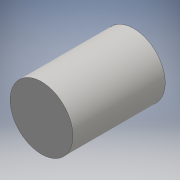
# Autodesk Inventor part: HarmonicDrive1
Saved by Autodesk Inventor 2016 (Build 200138000, 138)
## iProperties
Created: 2016-06-23
Part Number: HarmonicDrive1
Material: 一般
Document SubType Name: Modeling
Designer: 宏太
Density: 1 g/cm^3
Appearance: 既定
Author: 宏太
Autodesk Inventor part; units mm, degrees
ref_plane "YZ Plane" through (0, 0, 0) normal (1, 0, 0) x (0, 1, 0)
ref_plane "XZ Plane" through (0, 0, 0) normal (0, 1, 0) x (-1, 0, 0)
ref_plane "XY Plane" through (0, 0, 0) normal (0, 0, 1) x (1, 0, 0)
sketch "スケッチ1" plane through (0, 0, 0) normal (0, 1, 0) x (-1, 0, 0)
  circle A0 centre (0, 0) radius 20
  dimension "d0" = 40
  constraints: 1 centre point, 1 coincident
  measures "d0" diameter of A0
extrude "押し出し1" add sketch "スケッチ1" along normal blind 58.7
sketch "スケッチ2" plane through (0, 58.7, 0) normal (0, 1, 0) x (1, 0, 0)
  circle A0 centre (0, 0) radius 12
  dimension "d3" = 24
  constraints: 1 centre point, 1 coincident
  measures "d3" diameter of A0
extrude "押し出し2" add sketch "スケッチ2" along normal blind 3
hole "穴1" at (11.3305, 58.7, -10.9462) direction (0, -1, 0) diameter 4 depth 7
hole "穴2" at (-10.866, 58.7, 12.1709) direction (0, -1, 0) diameter 4 depth 7
hole "穴3" at (-11.4749, 58.7, -10.9538) direction (0, -1, 0) diameter 4 depth 7
hole "穴4" at (11.3606, 58.7, 10.8461) direction (0, -1, 0) diameter 4 depth 7
